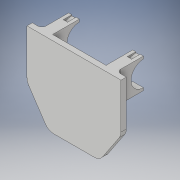
# Autodesk Inventor part: 7-8 HandlebarPlate
Saved by Autodesk Inventor 2019.1 (Build 231200000, 200)
## iProperties
Created: 2018-10-31
Part Number: 7-8 HandlebarPlate
Material: Generic
Document SubType Name: Modeling
Designer: eroldan
Density: 1 g/cm^3
Appearance: Default
Author: eroldan
Autodesk Inventor part; units mm, degrees
ref_plane "YZ Plane" through (0, 0, 0) normal (1, 0, 0) x (0, 1, 0)
ref_plane "XZ Plane" through (0, 0, 0) normal (0, 1, 0) x (-1, 0, 0)
ref_plane "XY Plane" through (0, 0, 0) normal (0, 0, 1) x (1, 0, 0)
sketch "Sketch1" plane through (0, 0, 0) normal (0, 0, 1) x (1, 0, 0)
  line L0 (-44, 0) -> (44, 0)
  line L1 (-24, -75) -> (24, -75)
  line L2 (-44, 0) -> (-44, -45)
  line L3 (44, 0) -> (44, -45)
  line L4 (-44, -45) -> (-24, -75)
  line L5 (24, -75) -> (44, -45)
  point P0 (0, 0)
  point P1 (0, 0)
  point P2 (0, -75)
  dimension "d0" = 88
  dimension "d1" = 48
  dimension "d2" = 75
  dimension "d4" = 45
  constraints: 12 end point, 2 horizontal, 2 midpoint, 2 vertical, 1 coincident, 1 horizontal alignment, 1 vertical alignment
  measures "d0" distance of L0.start L0.end
  measures "d1" distance of L1.start L1.end
  measures "d2" distance between parallel lines of L1 L0
  measures "d4" distance of L0.start L2.end
extrude "Extrusion1" add sketch "Sketch1" along normal blind 5
sketch "Sketch2" plane through (0, 0, 0) normal (0, 0, -1) x (-1, 0, 0)
  line L0 (-25, 0) -> (25, 0) construction
  line L1 (44, 0) -> (-44, 0) projected
  line L2 (-25, 0) -> (-35, 0)
  line L3 (-35, 0) -> (-35, -28)
  line L4 (-35, -28) -> (-25, -28)
  line L5 (-25, -28) -> (-25, 0)
  point P0 (0, 0)
  point P1 (0, 0)
  dimension "d7" = 50
  dimension "d8" = 10
  dimension "d9" = 28
  constraints: 10 end point, 2 horizontal, 2 midpoint, 2 parallel, 1 perpendicular
  measures "d7" distance of L0.start L0.end
  measures "d8" distance of L4.end L3.end
  measures "d9" distance of L3.end L2.end
extrude "Extrusion2" add sketch "Sketch2" along normal blind 25
sketch "Sketch3" plane through (25, -28, 0) normal (-1, 0, 0) x (0, 0, 1)
  line L0 (-25, 0) -> (-25, 28) projected
  circle A0 centre (-25, 14) radius 11.1125
  point P0 (0, 28)
  dimension "d12" = 22.225
  constraints: 1 centre point, 1 midpoint
  measures "d12" diameter of A0
extrude "Extrusion3" cut sketch "Sketch3" against normal through all
ref_plane "Work Plane1" through (30, -28, 0) normal (1, 0, 0) x (0, 0, -1)
sketch "Sketch4" plane through (30, -28, 0) normal (1, 0, 0) x (0, 0, -1)
  arc A0 (25, 25.1125) -> (25, 2.8875) centre (25, 14) ccw projected
  circle A1 centre (25, 14) radius 14.6312
  point P0 (0, 28)
  point P1 (25, -0.6312)
  point P2 (25, 28.6312)
  constraints: 2 point on circle, 1 centre point, 1 coincident
sketch "Sketch5" plane through (0, 0, -25) normal (0, 0, -1) x (-1, 0, 0)
  line L0 (-28, -27.1312) -> (-32, -27.1312)
  line L1 (-32, -27.1312) -> (-32, -30.1312)
  line L2 (-32, -30.1312) -> (-28, -30.1312)
  line L3 (-28, -30.1312) -> (-28, -27.1312)
  line L4 (-28, -27.1312) -> (-32, -30.1312) construction
  line L5 (-32, -27.1312) -> (-28, -30.1312) construction
  line L6 (61.6, -14) -> (-61.6, -14) projected
  point P0 (0, 0)
  point P1 (-30, -28.6312)
  dimension "d17" = 4
  dimension "d18" = 3
  constraints: 12 end point, 2 midpoint, 2 parallel, 1 horizontal, 1 perpendicular
  measures "d17" distance of L2.end L1.end
  measures "d18" distance of L1.end L0.end
revolve "Revolution1" cut sketch "Sketch5" angle 360 about axis through (30, -14, -25) along (1, 0, 0)
mirror "Mirror1" about plane through (0, 0, 0) normal (1, 0, 0) of "Extrusion2", "Extrusion3", "Revolution1"
fillet "Fillet1" radius 9.5 4 edges at (-24, -75, 2.5) (24, -75, 2.5) (44, -45, 2.5) (-44, -45, 2.5)
fillet "Fillet2" radius 3.75 4 edges at (35, -14, 0) (-35, -14, 0) (-30, -28, 0) (30, -28, 0)
thicken "Thicken1" operation add thickness 0.5 both sides no extend neighbours yes toward (0, -0.9485364, 0.316668) faces at (-28.3333, -24.5406, -21.481)
thicken "Thicken2" operation add thickness 0.5 both sides no extend neighbours yes toward (0, -0.8451901, 0.5344658) faces at (28.3333, -23.3922, -19.0607)
body "Solid1"
